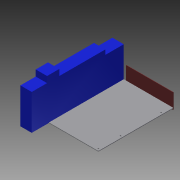
# Autodesk Inventor part: Mobo
Saved by Autodesk Inventor 2015 (Build 190159000, 159)
## iProperties
Created: 2016-03-23
Part Number: Mobo
Material: Generic
Document SubType Name: Modeling
Designer: Noah
Density: 1 g/cm^3
Appearance: Default
Author: Noah
Autodesk Inventor part; units mm, degrees
ref_plane "YZ Plane" through (0, 0, 0) normal (1, 0, 0) x (0, 1, 0)
ref_plane "XZ Plane" through (0, 0, 0) normal (0, 1, 0) x (-1, 0, 0)
ref_plane "XY Plane" through (0, 0, 0) normal (0, 0, 1) x (1, 0, 0)
sketch "Sketch1" plane through (0, 0, 0) normal (0, 0, 1) x (1, 0, 0)
  line L0 (-122, 122) -> (122, 122)
  line L1 (122, 122) -> (122, -122)
  line L2 (122, -122) -> (-122, -122)
  line L3 (-122, -122) -> (-122, 122)
  point P0 (0, 0)
  dimension "d0" = 244
  dimension "d1" = 244
  dimension "d2" = 122
  dimension "d3" = 122
  constraints: 8 end point, 2 parallel, 1 horizontal, 1 perpendicular
  measures "d0" distance of L0.end L1.end
  measures "d1" distance of L0.start L0.end
  measures "d2" distance from line of L0 point (0, 0)
  measures "d3" distance from line of L1 point (0, 0)
extrude "Extrusion1" add sketch "Sketch1" along normal blind 2
sketch "Sketch3" plane through (0, 0, 2) normal (0, 0, 1) x (1, 0, 0)
  line L0 (122, 122) -> (-122, 122) projected
  line L1 (-122, 122) -> (-122, -122) projected
  line L2 (-122, -122) -> (122, -122) projected
  line L3 (122, -122) -> (122, 122) projected
  line L4 (-209.7818, 111.84) -> (205.7988, 111.84) construction
  line L5 (-179.0523, -43.1) -> (193.3606, -43.1) construction
  line L6 (-192.2221, -115.49) -> (227.0168, -115.49) construction
  line L7 (115.49, -184.6971) -> (115.49, 232.3468) construction
  line L8 (-41.99, -199.0105) -> (-41.99, 288.2767) construction
  point P0 (0, 0)
  point P1 (-87.71, 111.84)
  point P2 (-41.99, 111.84)
  point P3 (-108.03, -43.1)
  point P4 (-87.71, -43.1)
  point P5 (-41.99, -43.1)
  point P6 (115.49, -43.1)
  point P7 (115.49, -115.49)
  point P8 (-41.99, -115.49)
  point P9 (115.49, 88.98)
  dimension "d12" = 34.29
  dimension "d13" = 20.32
  dimension "d18" = 10.16
  dimension "d20" = 227.33
  dimension "d22" = 90
  dimension "d23" = 22.86
  dimension "d24" = 154.94
  dimension "d25" = 45.72
  dimension "d26" = 203.2
  dimension "d27" = 45.72
  constraints: 14 point on line, 10 end point, 2 horizontal, 1 perpendicular, 1 vertical
  measures "d12" distance from line of L1 point (-87.71, -43.1)
  measures "d13" distance of point (-87.71, -43.1) point (-108.03, -43.1)
  measures "d18" distance from line of L0 point (-87.71, 111.84)
  measures "d20" distance between parallel lines of L6 L4
  measures "d22" angle of L5 L8
  measures "d23" distance from line of L4 point (115.49, 88.98)
  measures "d24" distance between parallel lines of L5 L4
  measures "d25" distance from line of L8 point (-87.71, -43.1)
  measures "d26" distance from line of L7 point (-87.71, -43.1)
  measures "d27" distance of point (-41.99, 111.84) point (-87.71, 111.84)
hole "Hole1" at (-87.71, 111.84, 2) at (-41.99, 111.84, 2) at (-108.03, -43.1, 2) at (-87.71, -43.1, 2) at (-41.99, -43.1, 2) at (115.49, -43.1, 2) at (115.49, -115.49, 2) at (-41.99, -115.49, 2) at (115.49, 88.98, 2) direction (0, 0, -1) diameter 3.96 end through all
fillet "Fillet1" radius 2 4 edges at (-122, 122, 1) (-122, -122, 1) (122, -122, 1) (122, 122, 1)
sketch "Sketch4" plane through (-120, 122, 0) normal (0, 1, 0) x (1, 0, 0)
  line L0 (34.27, -2) -> (30.31, -2) construction
  line L1 (32.29, -21.9524) -> (32.29, 25.1381) construction
  line L2 (241.79, -45.39) -> (87.79, -45.39)
  line L3 (87.79, -45.39) -> (87.79, 4.35)
  line L4 (87.79, 4.35) -> (241.79, 4.35)
  line L5 (241.79, 4.35) -> (241.79, -45.39)
  line L6 (240, -2) -> (0, -2) construction
  line L7 (34.27, -2) -> (30.31, -2) construction
  point P0 (120, 0)
  point P1 (32.29, -2)
  dimension "d36" = 154
  dimension "d37" = 49.74
  dimension "d38" = 55.5
  dimension "d39" = 6.35
  constraints: 10 end point, 2 parallel, 1 horizontal, 1 midpoint, 1 perpendicular, 1 point on line, 1 vertical
  measures "d36" distance of L3.end L4.end
  measures "d37" distance of L2.end L3.end
  measures "d38" distance between parallel lines of L1 L3
  measures "d39" distance between parallel lines of L4 L6
extrude "Extrusion3" add sketch "Sketch4" along normal blind 1.32
fillet "Fillet2" radius 1 4 edges at (121.79, 122.66, 45.39) (-32.21, 122.66, 45.39) (121.79, 122.66, -4.35) (-32.21, 122.66, -4.35)
sketch "Sketch5" plane through (-120, 122, 2) normal (0, 1, 0) x (1, 0, 0)
  line L0 (80.79, -98.65) -> (43.79, -98.65)
  line L1 (43.79, -98.65) -> (43.79, 1.35)
  line L2 (43.79, 1.35) -> (80.79, 1.35)
  line L3 (80.79, 1.35) -> (80.79, -98.65)
  line L4 (87.79, 5.35) -> (87.79, -42.39) projected
  line L5 (240.79, 6.35) -> (88.79, 6.35) projected
  point P0 (120, 2)
  dimension "d43" = 37
  dimension "d44" = 100
  dimension "d45" = 7
  dimension "d46" = 5
  constraints: 8 end point, 2 parallel, 1 horizontal, 1 perpendicular
  measures "d43" distance of L1.end L2.end
  measures "d44" distance of L0.end L1.end
  measures "d45" distance between parallel lines of L4 L3
  measures "d46" distance between parallel lines of L2 L5
extrude "Extrusion4" add sketch "Sketch5" against normal blind 300
sketch "Sketch7" plane through (-120, -178, 2) normal (0, -1, 0) x (1, 0, 0)
  line L0 (43.79, 114) -> (80.79, 114)
  line L1 (80.79, 114) -> (80.79, 0)
  line L2 (80.79, 0) -> (43.79, 0)
  line L3 (43.79, 0) -> (43.79, 114)
  point P0 (120, -2)
  dimension "d49" = 37
  dimension "d50" = 114
  constraints: 8 end point, 2 parallel, 1 horizontal, 1 perpendicular
  measures "d49" distance between parallel lines of L1 L3
  measures "d50" distance between parallel lines of L0 L2
extrude "Extrusion5" add sketch "Sketch7" against normal blind 240
sketch "Sketch8" plane through (-76.21, -178, 116) normal (0, 0, 1) x (1, 0, 0)
  line L0 (37, 0) -> (37, 240) projected
  line L1 (0, 0) -> (0, 240) projected
  line L2 (37, 90) -> (0, 90)
  line L3 (0, 90) -> (0, 50)
  line L4 (0, 50) -> (37, 50)
  line L5 (37, 50) -> (37, 90)
  line L6 (0, 0) -> (37, 0) projected
  point P0 (76.21, 178)
  dimension "d53" = 50
  dimension "d54" = 40
  constraints: 8 end point, 2 parallel, 2 point on line, 1 horizontal, 1 perpendicular
  measures "d53" distance between parallel lines of L6 L4
  measures "d54" distance between parallel lines of L4 L2
extrude "Extrusion6" add sketch "Sketch8" along normal blind 20 contours L4 L1 L2 L0
body "Solid1"
